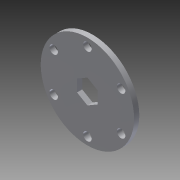
# Autodesk Inventor part: chassis hex hub clone
Saved by Autodesk Inventor 2014 SP1 (Build 180222100, 222)
## iProperties
Created: 2014-01-09
Part Number: chassis hex hub clone
Material: Aluminum 6061
Document SubType Name: Modeling
Designer: Arpan
Density: 2.71 g/cm^3
Appearance: Aluminum - Flat
Author: Arpan
Autodesk Inventor part; units mm, degrees
ref_plane "YZ Plane" through (0, 0, 0) normal (1, 0, 0) x (0, 1, 0)
ref_plane "XZ Plane" through (0, 0, 0) normal (0, 1, 0) x (-1, 0, 0)
ref_plane "XY Plane" through (0, 0, 0) normal (0, 0, 1) x (1, 0, 0)
sketch "Sketch1" plane through (0, 0, 0) normal (0, 0, 1) x (1, 0, 0)
  circle A0 centre (0, 0) radius 28.575
  line L0 (0, -7.3617) -> (6.3754, -3.6809)
  line L1 (-6.3754, -3.6809) -> (0, -7.3617)
  line L2 (-6.3754, 3.6808) -> (-6.3754, -3.6809)
  line L3 (0, 7.3617) -> (-6.3754, 3.6808)
  line L4 (6.3754, 3.6808) -> (0, 7.3617)
  line L5 (6.3754, -3.6809) -> (6.3754, 3.6808)
  circle A1 centre (0, 23.8125) radius 2.5908
  circle A2 centre (-20.6222, 11.9062) radius 2.5908
  circle A3 centre (-20.6222, -11.9062) radius 2.5908
  circle A4 centre (0, -23.8125) radius 2.5908
  circle A5 centre (20.6222, -11.9063) radius 2.5908
  circle A6 centre (20.6222, 11.9062) radius 2.5908
  arc A7 (-2.587, 23.6716) -> (-19.2067, 14.0762) centre (0, 0) ccw
  arc A8 (-21.7937, 9.5954) -> (-21.7937, -9.5954) centre (0, 0) ccw
  arc A9 (-19.2067, -14.0762) -> (-2.587, -23.6716) centre (0, 0) ccw
  arc A10 (2.587, -23.6716) -> (19.2067, -14.0762) centre (0, 0) ccw
  arc A11 (21.7937, -9.5954) -> (21.7937, 9.5954) centre (0, 0) ccw
  arc A12 (19.2067, 14.0762) -> (2.587, 23.6716) centre (0, 0) ccw
  dimension "d7" = 5.1816
  dimension "d12" = 360
  constraints: 24 point on circle, 13 centre point, 12 end point, 1 coincident, 25 other
  measures "d7" diameter of A1
extrude "Extrusion1" add sketch "Sketch1" along normal blind 3.175 contours A0 | A1 A12 A6 A11 A5 A10 A4 A9 A3 A8 A2 A7
body "Solid1"
